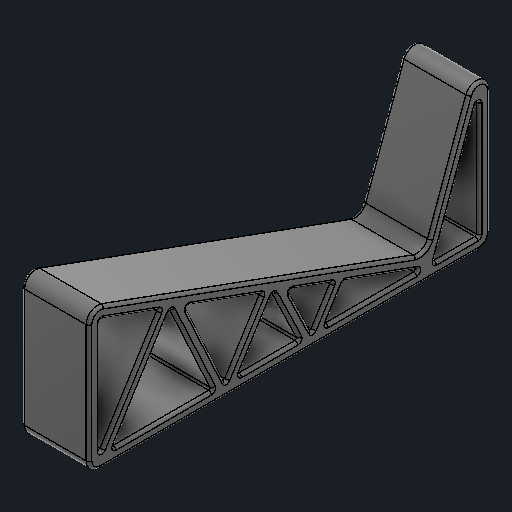
# Autodesk Inventor part: Cab Stand (25deg)
Saved by Autodesk Inventor 2026.2 (Build 302298000, 298)
## iProperties
Created: 2026-07-31
Part Number: Cab Stand (25deg)
Material: ABS Plastic
Document SubType Name: Modeling
Designer: JoshuaEah
Density: 1.06 g/cm^3
Appearance: Smooth - Black
Author: JoshuaEah
Autodesk Inventor part; units mm, degrees
ref_plane "YZ Plane" through (0, 0, 0) normal (1, 0, 0) x (0, 1, 0)
ref_plane "XZ Plane" through (0, 0, 0) normal (0, 1, 0) x (-1, 0, 0)
ref_plane "XY Plane" through (0, 0, 0) normal (0, 0, 1) x (1, 0, 0)
sketch "Sketch1" plane through (0, 0, 0) normal (1, 0, 0) x (0, 1, 0)
  line L0 (0, 0) -> (0, -227.1527)
  line L1 (0, 0) -> (82.1985, 0)
  line L2 (82.1985, 0) -> (12.7, -190.9455)
  line L3 (12.7, -190.9455) -> (84.3046, -217.0075)
  line L4 (84.3046, -217.0075) -> (80.612, -227.1527)
  line L5 (80.612, -227.1527) -> (0, -227.1527)
  line L6 (76.1657, -220.8027) -> (6.35, -195.3919)
  line L7 (6.35, -195.3919) -> (6.35, -220.8027)
  line L8 (6.35, -220.8027) -> (76.1657, -220.8027)
  line L9 (73.1298, -6.35) -> (6.35, -6.35)
  line L10 (6.35, -6.35) -> (60.7567, -40.3447)
  line L11 (60.7567, -40.3447) -> (73.1298, -6.35)
  line L12 (58.5364, -46.445) -> (6.35, -13.8376)
  line L13 (6.35, -13.8376) -> (6.35, -70.5445)
  line L14 (6.35, -70.5445) -> (58.5364, -46.445)
  line L15 (55.4763, -54.8526) -> (6.35, -77.5389)
  line L16 (55.4763, -54.8526) -> (39.6468, -98.3436)
  line L17 (39.6468, -98.3436) -> (6.35, -77.5389)
  line L18 (37.4265, -104.444) -> (6.35, -85.0266)
  line L19 (6.35, -85.0266) -> (6.35, -119.4484)
  line L20 (6.35, -119.4484) -> (37.4265, -104.444)
  line L21 (34.3128, -112.9987) -> (6.35, -126.4998)
  line L22 (6.35, -126.4998) -> (25.1283, -138.233)
  line L23 (25.1283, -138.233) -> (34.3128, -112.9987)
  line L24 (22.9079, -144.3333) -> (6.35, -133.9874)
  line L25 (6.35, -133.9874) -> (6.35, -189.8259)
  line L26 (6.35, -189.8259) -> (22.9079, -144.3333)
  point P0 (6.35, -195.4401)
  dimension "d1" = 203.2
  dimension "d2" = 76.2
  dimension "d12" = 6.35
  dimension "d13" = 6.35
  dimension "d14" = 6.35
  dimension "d15" = 12.7
  dimension "d16" = 6.35
  dimension "d24" = 20
  dimension "d25" = 6.35
  dimension "d26" = 6.35
  dimension "d27" = 6.35
  dimension "d28" = 6.35
  dimension "d29" = 6.35
  dimension "d32" = 6.35
  dimension "d34" = 6.35
  dimension "d35" = 6.35
  constraints: 54 end point, 15 point on line, 12 parallel, 3 horizontal, 3 perpendicular, 2 vertical, 1 coincident, 1 collinear
  measures "d1" distance of L1.end L2.end
  measures "d2" distance of L2.end L3.end
  measures "d12" distance between parallel lines of L3 L6
  measures "d13" distance between parallel lines of L5 L8
  measures "d14" distance between parallel lines of L0 L7
  measures "d15" distance from line of L0 L2.end
  measures "d16" distance from line of L4 L6.start
  measures "d24" angle of L0 L2
  measures "d25" distance between parallel lines of L2 L11
  measures "d26" distance between parallel lines of L1 L9
  measures "d27" distance between parallel lines of L12 L10
  measures "d28" distance between parallel lines of L15 L14
  measures "d29" distance between parallel lines of L0 L13
  measures "d32" distance between parallel lines of L17 L18
  measures "d34" distance between parallel lines of L22 L24
  measures "d35" distance between parallel lines of L21 L20
extrude "Extrusion1" add sketch "Sketch1" along normal blind 38.1
fillet "Fillet1" radius 6.35 6 edges at (19.05, 12.7, -190.9455) (19.05, 82.1985, 0) (19.05, 0, 0) (19.05, 0, -227.1527) (19.05, 80.612, -227.1527) (19.05, 84.3046, -217.0075)
fillet "Fillet1" radius 0.7937 21 edges at (19.05, 6.35, -195.3919) (19.05, 6.35, -220.8027) (19.05, 76.1657, -220.8027) (19.05, 73.1298, -6.35) (19.05, 6.35, -6.35) (19.05, 60.7567, -40.3447) (19.05, 58.5364, -46.445) (19.05, 6.35, -70.5445) (19.05, 6.35, -13.8376) (19.05, 55.4763, -54.8526) (19.05, 6.35, -77.5389) (19.05, 39.6468, -98.3436) (19.05, 37.4265, -104.444) (19.05, 6.35, -85.0266) (19.05, 6.35, -119.4484) (19.05, 6.35, -126.4998) (19.05, 25.1283, -138.233) (19.05, 34.3128, -112.9987) (19.05, 22.9079, -144.3333) (19.05, 6.35, -133.9874) (19.05, 6.35, -189.8259)
fillet "Fillet2" radius 1.5875 92 edges at (38.1, 72.4463, -220.1469) (38.1, 39.4042, -220.8027) (38.1, 6.5825, -220.5702) (38.1, 6.35, -208.2672) (38.1, 6.6884, -195.8752) (38.1, 39.6756, -207.5214) (0, 6.5825, -220.5702) (0, 6.35, -208.2672) (0, 6.6884, -195.8752) (0, 39.6756, -207.5214) (0, 72.4463, -220.1469) (0, 39.4042, -220.8027) (0, 78.3314, -2.7077) (0, 1.8598, -1.8598) (0, 1.8598, -225.2929) (0, 81.9208, -218.1191) (0, 79.8079, -226.0043) (0, 82.1328, -222.9745) (0, 30.7144, -66.2875) (38.1, 78.3314, -2.7077) (38.1, 1.8598, -1.8598) (38.1, 1.8598, -225.2929) (38.1, 81.9208, -218.1191) (38.1, 79.8079, -226.0043) (38.1, 82.1328, -222.9745) (38.1, 30.7144, -66.2875) (38.1, 6.716, -69.9724) (38.1, 6.35, -42.2866) (38.1, 6.7589, -14.5752) (38.1, 32.4277, -30.1317) (38.1, 57.6627, -46.39) (38.1, 32.3399, -58.5425) (0, 57.6627, -46.39) (0, 32.3399, -58.5425) (0, 6.716, -69.9724) (0, 6.35, -42.2866) (0, 6.7589, -14.5752) (0, 32.4277, -30.1317) (38.1, 60.6045, -39.9027) (38.1, 34.3115, -23.8211) (38.1, 8.355, -6.9249) (38.1, 40.5571, -6.35) (38.1, 72.6464, -6.6884) (38.1, 66.917, -23.4194) (0, 60.6045, -39.9027) (0, 34.3115, -23.8211) (0, 8.355, -6.9249) (0, 40.5571, -6.35) (0, 72.6464, -6.6884) (0, 66.917, -23.4194) (38.1, 6.7217, -118.8561) (38.1, 6.35, -102.3211) (38.1, 6.7589, -85.7642) (38.1, 21.8853, -94.7335) (38.1, 36.5784, -104.3978) (38.1, 21.8099, -111.984) (0, 21.8099, -111.984) (0, 6.7217, -118.8561) (0, 6.35, -102.3211) (0, 6.7589, -85.7642) (0, 21.8853, -94.7335) (0, 36.5784, -104.3978) (38.1, 39.4946, -97.9017) (38.1, 23.2054, -88.0706) (38.1, 47.4032, -77.0332) (0, 39.4946, -97.9017) (0, 23.2054, -88.0706) (0, 47.4032, -77.0332) (38.1, 24.9761, -137.791) (38.1, 15.9336, -132.4879) (38.1, 7.1981, -126.5459) (38.1, 20.0997, -119.8611) (38.1, 33.4312, -113.9739) (38.1, 29.5541, -126.0731) (0, 24.9761, -137.791) (0, 15.9336, -132.4879) (0, 7.1981, -126.5459) (0, 20.0997, -119.8611) (0, 33.4312, -113.9739) (0, 29.5541, -126.0731) (38.1, 7.0058, -186.1064) (38.1, 6.35, -160.372) (38.1, 6.7589, -134.725) (38.1, 14.9635, -139.3694) (38.1, 22.6927, -144.4074) (38.1, 15.2888, -165.2668) (0, 7.0058, -186.1064) (0, 6.35, -160.372) (0, 6.7589, -134.725) (0, 14.9635, -139.3694) (0, 22.6927, -144.4074) (0, 15.2888, -165.2668)
fillet_without_effect "Fillet3"
body "Solid1"
